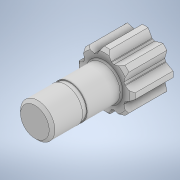
# Autodesk Inventor part: Shaft_stage_input_with_spline
Saved by Autodesk Inventor 2020 (Build 240168000, 168)
## iProperties
Created: 2020-05-12
Part Number: Shaft_stage_input_with_spline
Material: Generic
Document SubType Name: Modeling
Designer: avi41
Density: 1 g/cm^3
Appearance: Default
Author: avi41
Autodesk Inventor part; units mm, degrees
ref_plane "YZ Plane" through (0, 0, 0) normal (1, 0, 0) x (0, 1, 0)
ref_plane "XZ Plane" through (0, 0, 0) normal (0, 1, 0) x (-1, 0, 0)
sketch "Sketch1" plane through (0, 0, 0) normal (0, 1, 0) x (-1, 0, 0)
  line L0 (0, -13.475) -> (0, 13.475) construction
  line L1 (-6, 0) -> (1, 0) construction
  line L2 (0, 9.625) -> (-5, 9.625)
  line L3 (-5, 9.625) -> (-5, -9.625)
  line L4 (-5, -9.625) -> (0, -9.625)
  line L5 (0, 9.625) -> (0, -9.625)
  point P0 (0, 0)
  dimension "d0" = 5
  dimension "d1" = 19.25
  constraints: 8 end point, 3 perpendicular, 2 point on line, 1 horizontal, 1 other
  measures "d0" distance of L3.end L4.end
  measures "d1" distance of L2.end L3.end
revolve "Revolution1" add sketch "Sketch1" angle 360 about axis through (0, 0, 9.625) along (0, 0, -1)
ref_plane "Work Plane1" through (0, 0, -6.5) normal (0, 0, 1) x (1, 0, 0)
sketch "Sketch2" plane through (0, 0, 0) normal (0, 1, 0) x (-1, 0, 0)
  line L0 (5, -9.625) -> (-5, -9.625) construction
  line L1 (5, 9.625) -> (-5, 9.625) construction
  line L2 (0, -13.475) -> (0, 13.475) construction
  line L3 (-14, 0) -> (14, 0) construction
  line L4 (-5, -9.625) -> (-5, 9.625) projected
  line L5 (5, 9.625) -> (-5, 9.625) projected
  line L6 (-3, 9.625) -> (-3, -2.25)
  line L7 (-5, -2.5) -> (-5, 9.625)
  line L8 (-5, 9.625) -> (-3, 9.625)
  line L9 (-14, -6.5) -> (14, -6.5) projected
  line L10 (-5, -9.625) -> (-5, 9.625) projected
  line L11 (-5, 3.5) -> (-2.85, 3.5)
  line L12 (-2.85, 3.5) -> (-2.85, 4.3)
  line L13 (-2.85, 4.3) -> (-5, 4.3)
  line L14 (-5, 4.3) -> (-5, 3.5)
  line L15 (-5, -2.5) -> (-3.25, -2.5)
  arc A0 (-3.25, -2.5) -> (-3, -2.25) centre (-3.25, -2.25) ccw
  line L16 (-5, -2.5) -> (-5, -6.5)
  line L17 (-5, -9.625) -> (-5, 9.625) projected
  line L18 (-5, -6.5) -> (-6.625, -6.5)
  line L19 (-6.625, -6.5) -> (-6.625, -9.625)
  line L20 (5, -9.625) -> (-5, -9.625) projected
  point P0 (0, 0)
  point P1 (-10, -2.5)
  point P2 (-3, -7.625)
  point P3 (-3, 4.3)
  point P4 (-3, 3.5)
  point P5 (-4.5, -2.5)
  dimension "d34" = 0.8
  dimension "d35" = 2.85
  dimension "d40" = 0.25
  dimension "d44" = 4
  dimension "d45" = 6
  dimension "d46" = 3
  constraints: 22 end point, 6 point on line, 3 perpendicular, 2 parallel, 2 point on circle, 2 tangent, 1 centre point, 1 horizontal, 1 vertical, 2 other
  measures "d34" distance of L11.end L12.end
  measures "d35" distance between parallel lines of L2 L12
  measures "d40" radius of A0
  measures "d44" distance between parallel lines of L15 L9
  measures "d45" distance between parallel lines of L15 L11
  measures "d46" distance between parallel lines of L2 L6
revolve "Revolution2" cut sketch "Sketch2" angle 360 about axis through (0, 0, 0) along (0, 0, 1)
sketch "Sketch3" plane through (0, 0, -6.5) normal (0, 0, 1) x (1, 0, 0)
  circle A0 centre (0, 0) radius 5 construction
  line L0 (-7, 0) -> (7, 0) construction
  line L1 (0, 7) -> (0, -7) construction
  circle A1 centre (0, 0) radius 4.9 construction
  circle A2 centre (0, 0) radius 3.8 construction
  line L2 (-0.5, 4.8744) -> (-1.2405, 3.5918) construction
  line L3 (0.5, 4.8744) -> (1.2405, 3.5918) construction
  circle A3 centre (0, 0) radius 3.75 construction
  circle A4 centre (0, 0) radius 4.45 construction
  circle A5 centre (-1.3496, 3.7229) radius 0.16 construction
  circle A6 centre (1.3496, 3.7229) radius 0.16 construction
  circle A7 centre (0, 0) radius 3.8
  line L4 (0.5, 4.8744) -> (1.2405, 3.5918)
  line L5 (-0.5, 4.8744) -> (-1.2405, 3.5918)
  arc A8 (-1.2951, 3.5725) -> (-1.211, 3.6429) centre (-1.3496, 3.7229) ccw
  arc A9 (1.211, 3.6429) -> (1.2951, 3.5725) centre (1.3496, 3.7229) ccw
  arc A10 (0.5, 4.8744) -> (-0.5, 4.8744) centre (0, 0) ccw
  circle A11 centre (0, 0) radius 3.8 construction
  circle A12 centre (0, 0) radius 3.8
  circle A13 centre (0, 0) radius 4.45 construction
  circle A14 centre (0, 0) radius 3.75 construction
  circle A15 centre (0, 0) radius 4.9 construction
  arc A16 (-1.7196, 3.4323) -> (-1.6104, 3.4419) centre (-1.6782, 3.5868) ccw
  circle A17 centre (-1.6782, 3.5868) radius 0.16 construction
  arc A18 (-3.0932, 3.8003) -> (-3.8003, 3.0932) centre (0, 0) ccw
  line L6 (-3.0932, 3.8003) -> (-1.6626, 3.417) construction
  line L7 (-3.0932, 3.8003) -> (-1.6626, 3.417)
  line L8 (-3.8003, 3.0932) -> (-3.417, 1.6626) construction
  line L9 (-3.8003, 3.0932) -> (-3.417, 1.6626)
  arc A19 (-3.4419, 1.6104) -> (-3.4323, 1.7196) centre (-3.5868, 1.6782) ccw
  circle A20 centre (-3.5868, 1.6782) radius 0.16 construction
  circle A21 centre (0, 0) radius 3.8 construction
  circle A22 centre (0, 0) radius 3.8
  circle A23 centre (0, 0) radius 4.45 construction
  circle A24 centre (0, 0) radius 3.75 construction
  circle A25 centre (0, 0) radius 4.9 construction
  arc A26 (-3.6429, 1.211) -> (-3.5725, 1.2951) centre (-3.7229, 1.3496) ccw
  circle A27 centre (-3.7229, 1.3496) radius 0.16 construction
  arc A28 (-4.8744, 0.5) -> (-4.8744, -0.5) centre (0, 0) ccw
  line L10 (-4.8744, 0.5) -> (-3.5918, 1.2405) construction
  line L11 (-4.8744, 0.5) -> (-3.5918, 1.2405)
  line L12 (-4.8744, -0.5) -> (-3.5918, -1.2405) construction
  line L13 (-4.8744, -0.5) -> (-3.5918, -1.2405)
  arc A29 (-3.5725, -1.2951) -> (-3.6429, -1.211) centre (-3.7229, -1.3496) ccw
  circle A30 centre (-3.7229, -1.3496) radius 0.16 construction
  circle A31 centre (0, 0) radius 3.8 construction
  circle A32 centre (0, 0) radius 3.8
  circle A33 centre (0, 0) radius 4.45 construction
  circle A34 centre (0, 0) radius 3.75 construction
  circle A35 centre (0, 0) radius 4.9 construction
  arc A36 (-3.4323, -1.7196) -> (-3.4419, -1.6104) centre (-3.5868, -1.6782) ccw
  circle A37 centre (-3.5868, -1.6782) radius 0.16 construction
  arc A38 (-3.8003, -3.0932) -> (-3.0932, -3.8003) centre (0, 0) ccw
  line L14 (-3.8003, -3.0932) -> (-3.417, -1.6626) construction
  line L15 (-3.8003, -3.0932) -> (-3.417, -1.6626)
  line L16 (-3.0932, -3.8003) -> (-1.6626, -3.417) construction
  line L17 (-3.0932, -3.8003) -> (-1.6626, -3.417)
  arc A39 (-1.6104, -3.4419) -> (-1.7196, -3.4323) centre (-1.6782, -3.5868) ccw
  circle A40 centre (-1.6782, -3.5868) radius 0.16 construction
  circle A41 centre (0, 0) radius 3.8 construction
  circle A42 centre (0, 0) radius 3.8
  circle A43 centre (0, 0) radius 4.45 construction
  circle A44 centre (0, 0) radius 3.75 construction
  circle A45 centre (0, 0) radius 4.9 construction
  arc A46 (-1.211, -3.6429) -> (-1.2951, -3.5725) centre (-1.3496, -3.7229) ccw
  circle A47 centre (-1.3496, -3.7229) radius 0.16 construction
  arc A48 (-0.5, -4.8744) -> (0.5, -4.8744) centre (0, 0) ccw
  line L18 (-0.5, -4.8744) -> (-1.2405, -3.5918) construction
  line L19 (-0.5, -4.8744) -> (-1.2405, -3.5918)
  line L20 (0.5, -4.8744) -> (1.2405, -3.5918) construction
  line L21 (0.5, -4.8744) -> (1.2405, -3.5918)
  arc A49 (1.2951, -3.5725) -> (1.211, -3.6429) centre (1.3496, -3.7229) ccw
  circle A50 centre (1.3496, -3.7229) radius 0.16 construction
  circle A51 centre (0, 0) radius 3.8 construction
  circle A52 centre (0, 0) radius 3.8
  circle A53 centre (0, 0) radius 4.45 construction
  circle A54 centre (0, 0) radius 3.75 construction
  circle A55 centre (0, 0) radius 4.9 construction
  arc A56 (1.7196, -3.4323) -> (1.6104, -3.4419) centre (1.6782, -3.5868) ccw
  circle A57 centre (1.6782, -3.5868) radius 0.16 construction
  arc A58 (3.0932, -3.8003) -> (3.8003, -3.0932) centre (0, 0) ccw
  line L22 (3.0932, -3.8003) -> (1.6626, -3.417) construction
  line L23 (3.0932, -3.8003) -> (1.6626, -3.417)
  line L24 (3.8003, -3.0932) -> (3.417, -1.6626) construction
  line L25 (3.8003, -3.0932) -> (3.417, -1.6626)
  arc A59 (3.4419, -1.6104) -> (3.4323, -1.7196) centre (3.5868, -1.6782) ccw
  circle A60 centre (3.5868, -1.6782) radius 0.16 construction
  circle A61 centre (0, 0) radius 3.8 construction
  circle A62 centre (0, 0) radius 3.8
  circle A63 centre (0, 0) radius 4.45 construction
  circle A64 centre (0, 0) radius 3.75 construction
  circle A65 centre (0, 0) radius 4.9 construction
  arc A66 (3.6429, -1.211) -> (3.5725, -1.2951) centre (3.7229, -1.3496) ccw
  circle A67 centre (3.7229, -1.3496) radius 0.16 construction
  arc A68 (4.8744, -0.5) -> (4.8744, 0.5) centre (0, 0) ccw
  line L26 (4.8744, -0.5) -> (3.5918, -1.2405) construction
  line L27 (4.8744, -0.5) -> (3.5918, -1.2405)
  line L28 (4.8744, 0.5) -> (3.5918, 1.2405) construction
  line L29 (4.8744, 0.5) -> (3.5918, 1.2405)
  arc A69 (3.5725, 1.2951) -> (3.6429, 1.211) centre (3.7229, 1.3496) ccw
  circle A70 centre (3.7229, 1.3496) radius 0.16 construction
  circle A71 centre (0, 0) radius 5
  circle A72 centre (0, 0) radius 3.8 construction
  circle A73 centre (0, 0) radius 3.8
  circle A74 centre (0, 0) radius 4.45 construction
  circle A75 centre (0, 0) radius 3.75 construction
  circle A76 centre (0, 0) radius 4.9 construction
  arc A77 (3.4323, 1.7196) -> (3.4419, 1.6104) centre (3.5868, 1.6782) ccw
  circle A78 centre (3.5868, 1.6782) radius 0.16 construction
  arc A79 (3.8003, 3.0932) -> (3.0932, 3.8003) centre (0, 0) ccw
  line L30 (3.8003, 3.0932) -> (3.417, 1.6626) construction
  line L31 (3.8003, 3.0932) -> (3.417, 1.6626)
  line L32 (3.0932, 3.8003) -> (1.6626, 3.417) construction
  line L33 (3.0932, 3.8003) -> (1.6626, 3.417)
  arc A80 (1.6104, 3.4419) -> (1.7196, 3.4323) centre (1.6782, 3.5868) ccw
  circle A81 centre (1.6782, 3.5868) radius 0.16 construction
  point P0 (-0.7854, 4.3801)
  point P1 (0.7854, 4.3801)
  point P2 (-3.6526, 2.5419)
  point P3 (-2.5419, 3.6526)
  point P4 (-4.3801, -0.7854)
  point P5 (-4.3801, 0.7854)
  point P6 (-2.5419, -3.6526)
  point P7 (-3.6526, -2.5419)
  point P8 (0.7854, -4.3801)
  point P9 (-0.7854, -4.3801)
  point P10 (3.6526, -2.5419)
  point P11 (2.5419, -3.6526)
  point P12 (4.3801, 0.7854)
  point P13 (4.3801, -0.7854)
  point P14 (3.5725, 1.2951)
  point P15 (3.5725, -1.2951)
  point P16 (3.4419, -1.6104)
  point P17 (1.6104, -3.4419)
  point P18 (1.2951, -3.5725)
  point P19 (-1.2951, -3.5725)
  point P20 (-1.6104, -3.4419)
  point P21 (-3.4419, -1.6104)
  point P22 (-3.5725, 1.2951)
  point P23 (-1.6104, 3.4419)
  point P24 (2.5419, 3.6526)
  point P25 (3.6526, 2.5419)
  point P26 (1.6626, 3.417)
  point P27 (3.417, 1.6626)
  dimension "d8" = 9.8
  dimension "d9" = 7.6
  dimension "d11" = 7.5
  dimension "d12" = 0.65
  dimension "d13" = 1.5708
  dimension "d14" = 0.32
  dimension "d21" = 360
  dimension "d29" = 30
  constraints: 112 point on circle, 82 centre point, 64 end point, 57 coincident, 32 point on line, 4 concentric, 3 tangent, 1 collinear, 1 symmetric about line, 274 other
  measures "d8" diameter of A1
  measures "d9" diameter of A2
  measures "d11" diameter of A3
  measures "d12" radial gap between concentric circles of A4 A2
  measures "d13" distance of A4.end A4.start
  measures "d14" diameter of A5
  measures "d29" angle of L2 L1
extrude "Extrusion1" cut sketch "Sketch3" along normal through all both and the other way through all contours A7 L31 A77 | A7 A80 L33 | A71
chamfer "Chamfer1" distance 0.5 angle 45 8 edges at (3.4648, 3.4648, -2.5) (0, 4.9, -2.5) (-3.4648, 3.4648, -2.5) (-4.9, 0, -2.5) (-3.4648, -3.4648, -2.5) (0, -4.9, -2.5) (3.4648, -3.4648, -2.5) (4.9, 0, -2.5)
chamfer "Chamfer2" distance 0.5 angle 45 1 edges at (-3, 0, 9.625)
equation "\"d8\" = tip_circ_diam_shaft"
equation "\"d9\" = root_circ_diam_shaft"
equation "\"d11\" = base_form_circ_diam_shaft"
equation "\"d12\" = dedendum"
equation "\"d13\" = 0.5 * pitch"
equation "\"d14\" = 2 * root_fillet_r"
equation "\"module\" = 1"
equation "\"pressure_ang\" = 30deg"
equation "\"pitch\" = 3.1416 * module"
equation "\"addendum\" = 0.45 * module"
equation "\"dedendum\" = 0.65 * module"
equation "\"tooth_depth\" = addendum + dedendum"
equation "\"addendum_mod_shaft\" = 0.45 * module"
equation "\"root_fillet_r\" = 0.16 * module"
equation "\"addendum_mod_hub\" = -addendum_mod_shaft"
equation "\"nom_space_t_hub\" = nom_tooth_t_shaft"
equation "\"tip_circ_diam_shaft\" = 9.8"
equation "\"root_circ_diam_shaft\" = 7.6"
equation "\"base_form_circ_diam_shaft\" = 7.5"
equation "\"nom_tooth_t_shaft\" = 2.090415"
body "Solid1"
